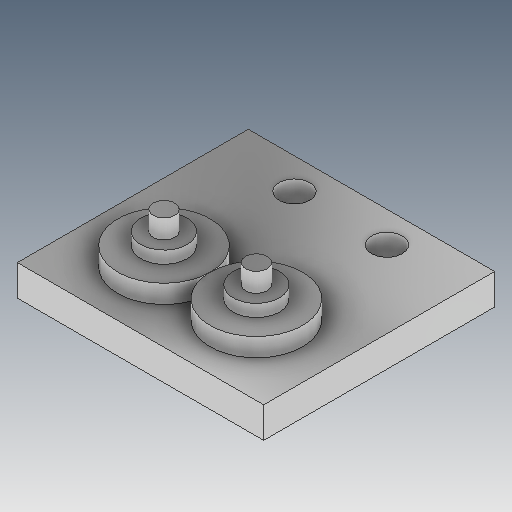
# Autodesk Inventor part: Gripping Claws
Saved by Autodesk Inventor 2021 (Build 250183000, 183)
## iProperties
Created: 2021-06-21
Part Number: Gripping Claws
Material: Nickel-Copper Alloy 400
Document SubType Name: Modeling
Designer: dell
Density: 8.83 g/cm^3
Appearance: Chrome - Polished
Author: dell
Autodesk Inventor part; units mm, degrees
ref_plane "YZ Plane" through (0, 0, 0) normal (1, 0, 0) x (0, 1, 0)
ref_plane "XZ Plane" through (0, 0, 0) normal (0, 1, 0) x (-1, 0, 0)
ref_plane "XY Plane" through (0, 0, 0) normal (0, 0, 1) x (1, 0, 0)
sketch "Sketch9" plane through (0, 0, 0) normal (0, 1, 0) x (-1, 0, 0)
  line L0 (0, 0) -> (127, 0)
  line L1 (127, 0) -> (127, -127)
  line L2 (127, -127) -> (0, -127)
  line L3 (0, -127) -> (0, 0)
  dimension "d29" = 127
  dimension "d30" = 127
  constraints: 8 end point, 2 parallel, 1 horizontal, 1 perpendicular
  measures "d29" distance of L1.end L2.end
  measures "d30" distance of L0.end L1.end
extrude "Extrusion9" add sketch "Sketch9" along normal blind 12.7
sketch "Sketch10" plane through (0, 12.7, 0) normal (0, 1, 0) x (1, 0, 0)
  line L0 (-127, 127) -> (-127, 0) projected
  line L1 (-127, 0) -> (0, 0) projected
  line L2 (0, 0) -> (0, 127) projected
  line L3 (0, 127) -> (-127, 127) projected
  circle A0 centre (-88.9, 50.8) radius 19.05
  circle A1 centre (-38.1, 50.8) radius 19.05
  circle A2 centre (-82.55, 101.6) radius 6.35
  circle A3 centre (-44.45, 101.6) radius 6.35
  point P0 (-38.1, 101.6)
  constraints: 4 centre point, 1 coincident
extrude "Extrusion10" cut sketch "Sketch10" against normal through all contours A2 | A3
sketch "Sketch11" plane through (0, 12.7, 0) normal (0, 1, 0) x (1, 0, 0)
  circle A0 centre (-82.55, 47.7782) radius 19.05
  circle A1 centre (-44.45, 101.6) radius 6.35 projected
  line L0 (-127, 0) -> (0, 0) projected
  circle A2 centre (-44.45, 47.7782) radius 19.05
  line L1 (-44.45, 101.6) -> (-44.45, 95.25)
  point P0 (-63.5, 47.7782)
  dimension "d47" = 38.1
  dimension "d48" = 38.1
  constraints: 2 centre point, 2 end point, 1 vertical, 1 vertical alignment, 1 other
  measures "d47" diameter of A0
  measures "d48" diameter of A2
extrude "Extrusion11" add sketch "Sketch11" along normal blind 7.62 contours A0 | A2
sketch "Sketch12" plane through (-127, 0, 0) normal (0, 0, 1) x (1, 0, 0)
  line L0 (0, 0) -> (0, 12.7) projected
  line L1 (127, 0) -> (0, 0) projected
  line L2 (0, 12.7) -> (127, 12.7)
  line L3 (127, 12.7) -> (127, 0)
  line L4 (127, 0) -> (0, 0)
  line L5 (0, 0) -> (0, 12.7)
  constraints: 8 end point, 2 parallel, 1 horizontal, 1 perpendicular
extrude "Extrusion12" cut sketch "Sketch12" against normal blind 19.05
sketch "Sketch13" plane through (0, 0, -127) normal (0, 0, -1) x (-1, 0, 0)
  line L0 (0, 12.7) -> (127, 12.7) projected
  line L1 (127, 0) -> (127, 12.7) projected
  line L2 (0, 12.7) -> (127, 12.7)
  line L3 (127, 12.7) -> (127, 0)
  line L4 (127, 0) -> (0, 0)
  line L5 (0, 0) -> (0, 12.7)
  constraints: 8 end point, 2 parallel, 1 horizontal, 1 perpendicular
extrude "Extrusion13" cut sketch "Sketch13" against normal blind 12.7
sketch "Sketch14" plane through (-127, 0, -19.05) normal (-1, 0, 0) x (0, 0, 1)
  line L0 (-95.25, 12.7) -> (0, 12.7) projected
  line L1 (-95.25, 0) -> (0, 0) projected
  line L2 (-95.25, 12.7) -> (0, 12.7)
  line L3 (0, 12.7) -> (0, 0)
  line L4 (0, 0) -> (-95.25, 0)
  line L5 (-95.25, 0) -> (-95.25, 12.7)
  point P0 (19.05, 0)
  point P1 (0, 12.7)
  constraints: 8 end point, 2 parallel, 1 horizontal, 1 perpendicular
extrude "Extrusion14" cut sketch "Sketch14" against normal blind 12.7
sketch "Sketch15" plane through (0, 0, -19.05) normal (1, 0, 0) x (0, 0, -1)
  line L0 (0, 12.7) -> (0, 0) projected
  line L1 (95.25, 0) -> (95.25, 12.7) projected
  line L2 (0, 12.7) -> (95.25, 12.7)
  line L3 (95.25, 12.7) -> (95.25, 0)
  line L4 (95.25, 0) -> (0, 0)
  line L5 (0, 0) -> (0, 12.7)
  point P0 (-19.05, 0)
  constraints: 8 end point, 2 parallel, 1 horizontal, 1 perpendicular
extrude "Extrusion15" cut sketch "Sketch15" against normal blind 12.7
sketch "Sketch16" plane through (-44.45, 20.32, -47.7782) normal (0, 1, 0) x (1, 0, 0)
  circle A0 centre (0, 0) radius 9.525
  point P0 (44.45, -47.7782)
  dimension "d59" = 19.05
  constraints: 1 centre point
  measures "d59" diameter of A0
extrude "Extrusion16" add sketch "Sketch16" along normal blind 5.08
sketch "Sketch17" plane through (-82.55, 20.32, -47.7782) normal (0, 1, 0) x (1, 0, 0)
  circle A0 centre (0, 0) radius 9.525
  point P0 (82.55, -47.7782)
  dimension "d62" = 19.05
  constraints: 1 centre point
  measures "d62" diameter of A0
extrude "Extrusion17" add sketch "Sketch17" along normal blind 5.08
sketch "Sketch18" plane through (-44.45, 25.4, -47.7782) normal (0, 1, 0) x (1, 0, 0)
  circle A0 centre (0, 0) radius 4.445
  circle A1 centre (-38.1, 0) radius 19.05 projected
  circle A2 centre (-38.1, 0) radius 4.445
  point P0 (44.45, -47.7782)
  point P1 (-19.05, 0)
  dimension "d65" = 8.89
  dimension "d66" = 8.89
  constraints: 2 centre point, 1 coincident, 1 horizontal alignment
  measures "d65" diameter of A0
  measures "d66" diameter of A2
extrude "Extrusion18" add sketch "Sketch18" along normal blind 7.874 contours A0 | A2
body "Solid2"
